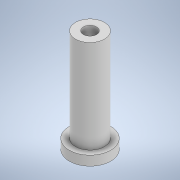
# Autodesk Inventor part: unwind_roller
Saved by Autodesk Inventor 2021 (Build 250183000, 183)
## iProperties
Created: 2024-02-27
Part Number: unwind_roller
Material: Generic
Document SubType Name: Modeling
Designer: Sebastián
Density: 1 g/cm^3
Appearance: Default
Author: Sebastián
Autodesk Inventor part; units mm, degrees
ref_plane "YZ Plane" through (0, 0, 0) normal (1, 0, 0) x (0, 1, 0)
ref_plane "XZ Plane" through (0, 0, 0) normal (0, 1, 0) x (-1, 0, 0)
ref_plane "XY Plane" through (0, 0, 0) normal (0, 0, 1) x (1, 0, 0)
sketch "Sketch1" plane through (0, 0, 0) normal (1, 0, 0) x (0, 1, 0)
  line L0 (-20.2, 10) -> (-24.8, 10)
  line L1 (-24.8, 10) -> (-24.8, 3.2)
  line L2 (20.2, 7) -> (-20.2, 7)
  line L3 (-20.2, 7) -> (-20.2, 10)
  line L4 (0, 12) -> (0, -2) construction
  line L5 (-34.72, 0) -> (34.72, 0) construction
  line L6 (-24.8, 3.2) -> (24.8, 3.2)
  line L7 (24.8, 3.2) -> (24.8, 7)
  line L8 (24.8, 7) -> (20.2, 7)
  point P0 (0, 0)
  dimension "d5" = 40.4
  dimension "d12" = 3
  dimension "d13" = 10
  dimension "d14" = 3.2
  constraints: 14 end point, 3 perpendicular, 1 horizontal, 1 parallel, 1 symmetric about line, 1 vertical
  measures "d5" distance of L2.start L2.end
  measures "d12" distance of L2.end L0.start
  measures "d13" distance from line of L5 L0.end
  measures "d14" distance from line of L5 L1.end
revolve "Revolution1" add sketch "Sketch1" angle 360 about axis through (0, 0, 0) along (0, 1, 0)
body "Solid1"
